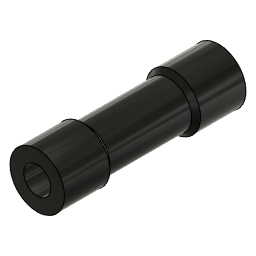
frame_assy (Autodesk Fusion 360 archive; units mm, degrees)
design "m3_standoff_20mm"
Autodesk Fusion 360 part; units mm, degrees
(part 1 of 5)
sketch "Sketch1" plane through (0, 0, 0) normal (0, 1, 0) x (1, 0, 0)
  line L0 (0, 0) -> (0, 20) construction
  line L1 (0, 20) -> (1.5, 20)
  line L2 (1.5, 20) -> (1.5, -8)
  line L3 (1.5, -8) -> (0, -8)
  line L4 (0, -8) -> (0, 20)
  line L5 (0, 20) -> (3, 20)
  line L6 (3, 20) -> (3, 15)
  line L7 (3, 15) -> (0, 15)
  line L8 (0, 15) -> (0, 20)
  line L9 (0, 0) -> (3, 0)
  line L10 (3, 0) -> (3, 5)
  line L11 (3, 5) -> (0, 5)
  line L12 (0, 5) -> (0, 0)
  line L13 (0, 15) -> (2.5, 15)
  line L14 (2.5, 15) -> (2.5, -3)
  line L15 (2.5, -3) -> (0, -3)
  line L16 (0, -3) -> (0, 15)
  dimension "d1" = 20
  dimension "d2" = 1.5
  dimension "d3" = 28
  dimension "d4" = 3
  dimension "d5" = 5
  dimension "d6" = 3
  dimension "d7" = 5
  dimension "d8" = 2.5
  constraint coincident L0.start L9.start
  constraint vertical L0
  constraint horizontal L1
  constraint vertical L2
  constraint horizontal L3
  constraint vertical L4
  constraint horizontal L5
  constraint vertical L6
  constraint horizontal L7
  constraint vertical L8
  constraint horizontal L9
  constraint vertical L10
  constraint horizontal L11
  constraint vertical L12
  constraint horizontal L13
  constraint vertical L14
  constraint horizontal L15
  constraint vertical L16
  measures "d1" distance of L0.start L0.end
  measures "d2" distance of L0.end L1.end
  measures "d3" distance of L0.end L3.end
  measures "d4" distance of L0.end L5.end
  measures "d5" distance of L0.end L7.end
  measures "d6" distance of L0.start L9.end
  measures "d7" distance of L0.start L11.end
  measures "d8" distance of L7.end L13.end
revolve "Revolve1" add sketch "Sketch1" angle 360 about axis through (0, 0, 3) along (0, 0, -1) contours L2 L5 L6 L7 L13 | L2 L7 L11 L13 L14 | L2 L9 L11 L14 | L9 L10 L11 L14
chamfer "Chamfer1" distance 0.5 angle 45 2 edges at (-2.3308, -0.904, -15) (-2.3308, -0.904, -5)

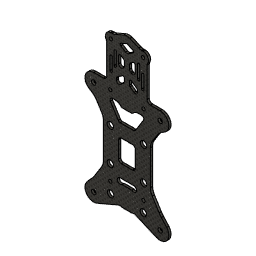
design "bottom_plate_2mm"
Autodesk Fusion 360 part; units mm, degrees
sketch "Sketch1" plane through (0, 0, 0) normal (0, 0, 1) x (1, 0, 0)
  line L0 (0, 26.674) -> (0, -149.1667) construction
  line L1 (30.5, -37.4) -> (-30.5, -37.4) construction
  line L2 (-30.5, -37.4) -> (-30.5, -124.4) construction
  line L3 (-30.5, -124.4) -> (30.5, -124.4) construction
  line L4 (30.5, -124.4) -> (30.5, -37.4) construction
  line L5 (30.5, -37.4) -> (-30.5, -124.4) construction
  line L6 (-30.5, -37.4) -> (30.5, -124.4) construction
  line L7 (-15.25, -63.8) -> (15.25, -63.8) construction
  line L8 (15.25, -63.8) -> (15.25, -94.3) construction
  line L9 (15.25, -94.3) -> (-15.25, -94.3) construction
  line L10 (-15.25, -94.3) -> (-15.25, -63.8) construction
  line L11 (-15.25, -63.8) -> (15.25, -94.3) construction
  line L12 (15.25, -63.8) -> (-15.25, -94.3) construction
  line L13 (5.15, -89.2) -> (-5.15, -89.2)
  line L14 (-7.65, -86.7) -> (-7.65, -71.4)
  line L15 (-5.15, -68.9) -> (5.15, -68.9)
  line L16 (7.65, -71.4) -> (7.65, -86.7)
  line L17 (7.65, -89.2) -> (-7.65, -68.9) construction
  line L18 (-7.65, -89.2) -> (7.65, -68.9) construction
  circle A0 centre (14.75, 5.1) radius 1.5
  line L19 (0, 0) -> (0, 7.5) construction
  line L20 (0, 7.5) -> (0, 13.8) construction
  line L21 (18.55, 0.8857) -> (18.55, -26.4)
  line L22 (14.75, 10.1) -> (0, 10.1)
  line L23 (21.55, -29.4) -> (30.5, -29.4)
  circle A1 centre (15.25, -63.8) radius 2.95
  circle A2 centre (15.25, -94.3) radius 2.95
  circle A3 centre (-15.25, -94.3) radius 2.95
  circle A4 centre (-15.25, -63.8) radius 2.95
  line L24 (12.25, 10.1) -> (0, 15.4402)
  circle A5 centre (15.25, -35.5) radius 1.5
  arc A6 (18.55, -26.4) -> (21.55, -29.4) centre (21.55, -26.4) ccw
  line L25 (30.5, -37.4) -> (30.5, -29.4) construction
  circle A7 centre (30.5, -37.4) radius 8
  circle A8 centre (30.5, -37.4) radius 2
  circle A9 centre (30.5, -124.4) radius 2
  circle A10 centre (30.5, -124.4) radius 8
  arc A11 (-5.15, -68.9) -> (-7.65, -71.4) centre (-5.15, -71.4) ccw
  arc A12 (7.65, -71.4) -> (5.15, -68.9) centre (5.15, -71.4) ccw
  arc A13 (5.15, -89.2) -> (7.65, -86.7) centre (5.15, -86.7) ccw
  arc A14 (-7.65, -86.7) -> (-5.15, -89.2) centre (-5.15, -86.7) ccw
  arc A15 (19, 2.4661) -> (14.75, 10.1) centre (14.75, 5.1) ccw
  arc A16 (14.75, 10.1) -> (18.55, 1.8504) centre (14.75, 5.1) ccw
  arc A17 (19, 2.4661) -> (18.55, 0.8857) centre (21.55, 0.8857) ccw
  line L26 (21.55, -98.0838) -> (21.55, -90.0777)
  line L27 (21.55, -90.0777) -> (21.55, -60.0565)
  line L28 (21.55, -60.0565) -> (30.7101, -45.3972)
  line L29 (21.55, -60.0565) -> (38.6049, -60.0565) construction
  line L30 (21.55, -98.0838) -> (30.5, -112.4068)
  line L31 (21.55, -98.0838) -> (38.4394, -98.0838) construction
  line L32 (30.5, -112.4068) -> (36.4601, -119.0636)
  line L33 (0, -123.6) -> (4.5, -123.6)
  line L34 (4.5, -123.6) -> (8.3, -123.6) construction
  arc A18 (8.3, -123.6) -> (4.5, -123.6) centre (6.4, -126.96) ccw
  line L35 (6.4, -123.1) -> (6.4, -123.6) construction
  line L36 (8.3, -123.6) -> (27.3521, -131.7546)
  line L37 (15.25, -94.3) -> (15.25, -108.3) construction
  circle A19 centre (15.25, -108.3) radius 1.5
  circle A20 centre (15, -118.1) radius 2.95
  arc A21 (-18.55, 1.8504) -> (-14.75, 10.1) centre (-14.75, 5.1) ccw
  line L38 (-21.55, -60.0565) -> (-30.7101, -45.3972)
  line L39 (-18.55, 0.8857) -> (-18.55, -26.4)
  circle A22 centre (-15.25, -35.5) radius 1.5
  circle A23 centre (-30.5, -37.4) radius 2
  line L40 (-14.75, 10.1) -> (0, 10.1)
  line L41 (0, 0) -> (0, 7.5) construction
  line L42 (-21.55, -90.0777) -> (-21.55, -60.0565)
  circle A24 centre (-14.75, 5.1) radius 1.5
  line L43 (-15.25, -63.8) -> (-15.25, -94.3) construction
  line L44 (-21.55, -29.4) -> (-30.5, -29.4)
  line L45 (-7.65, -89.2) -> (7.65, -68.9) construction
  line L46 (0, 7.5) -> (0, 13.8) construction
  arc A25 (-14.75, 10.1) -> (-19, 2.4661) centre (-14.75, 5.1) ccw
  line L47 (-30.5, -124.4) -> (-30.5, -37.4) construction
  line L48 (-21.55, -98.0838) -> (-30.5, -112.4068)
  line L49 (-12.25, 10.1) -> (0, 15.4402)
  arc A26 (-18.55, 0.8857) -> (-19, 2.4661) centre (-21.55, 0.8857) ccw
  line L50 (0, -123.6) -> (-4.5, -123.6)
  circle A27 centre (-15.25, -63.8) radius 2.95
  circle A28 centre (-30.5, -37.4) radius 8
  arc A29 (-21.55, -29.4) -> (-18.55, -26.4) centre (-21.55, -26.4) ccw
  line L51 (-30.5, -37.4) -> (-30.5, -29.4) construction
  line L52 (-21.55, -98.0838) -> (-38.4394, -98.0838) construction
  circle A30 centre (-15.25, -94.3) radius 2.95
  line L53 (5.15, -68.9) -> (-5.15, -68.9)
  line L54 (-6.4, -123.1) -> (-6.4, -123.6) construction
  arc A31 (-5.15, -68.9) -> (-7.65, -71.4) centre (-5.15, -71.4) ccw
  line L55 (-21.55, -98.0838) -> (-21.55, -90.0777)
  line L56 (-7.65, -71.4) -> (-7.65, -86.7)
  arc A32 (7.65, -71.4) -> (5.15, -68.9) centre (5.15, -71.4) ccw
  arc A33 (5.15, -89.2) -> (7.65, -86.7) centre (5.15, -86.7) ccw
  arc A34 (-7.65, -86.7) -> (-5.15, -89.2) centre (-5.15, -86.7) ccw
  line L57 (7.65, -86.7) -> (7.65, -71.4)
  line L58 (7.65, -89.2) -> (-7.65, -68.9) construction
  line L59 (-21.55, -60.0565) -> (-38.6049, -60.0565) construction
  line L60 (-8.3, -123.6) -> (-27.3521, -131.7546)
  line L61 (-15.25, -94.3) -> (-15.25, -108.3) construction
  circle A35 centre (-15, -118.1) radius 2.95
  line L62 (-30.5, -112.4068) -> (-36.4601, -119.0636)
  line L63 (-4.5, -123.6) -> (-8.3, -123.6) construction
  circle A36 centre (-30.5, -124.4) radius 8
  arc A37 (-4.5, -123.6) -> (-8.3, -123.6) centre (-6.4, -126.96) ccw
  circle A38 centre (-15.25, -108.3) radius 1.5
  circle A39 centre (-30.5, -124.4) radius 2
  line L64 (-5.15, -89.2) -> (5.15, -89.2)
  point P0 (0, -80.9)
  point P1 (0, -79.05)
  point P2 (0, -79.05)
  point P3 (18.55, -29.4)
  point P4 (0, -149.1667)
  point P5 (0, -79.05)
  point P6 (0, 26.674)
  point P7 (-18.55, -29.4)
  point P8 (0, -79.05)
  point P9 (0, -80.9)
  dimension "d1" = 61
  dimension "d2" = 87
  dimension "d3" = 30.5
  dimension "d4" = 30.5
  dimension "d7" = 15.3
  dimension "d8" = 20.3
  dimension "d9" = 68.9
  dimension "d10" = 3
  dimension "d11" = 14.75
  dimension "d14" = 7.5
  dimension "d15" = 6.3
  dimension "d17" = 10
  dimension "d18" = 18.55
  dimension "d19" = 39.5
  dimension "d20" = 5.9
  dimension "d21" = 8.7
  dimension "d22" = 2.5
  dimension "d24" = 3
  dimension "d25" = 15.25
  dimension "d26" = 40.6
  dimension "d27" = 3
  dimension "d28" = 8
  dimension "d29" = 4
  dimension "d30" = 16
  dimension "d31" = 2.5
  dimension "d32" = 3
  dimension "d33" = 21.55
  dimension "d34" = 58
  dimension "d35" = 58
  dimension "d36" = 34.4
  dimension "d37" = 3.8
  dimension "d38" = 4.5
  dimension "d39" = 0.5
  dimension "d41" = 72.8
  dimension "d42" = 15
  dimension "d43" = 23.8
  constraint vertical L0
  constraint horizontal L1
  constraint perpendicular L1 L2
  constraint parallel L1 L3
  constraint parallel L2 L4
  constraint coincident L5 P9
  constraint coincident L6 P9
  constraint coincident L0 P9
  constraint horizontal L7
  constraint perpendicular L7 L8
  constraint parallel L7 L9
  constraint parallel L8 L10
  constraint coincident L11 P8
  constraint coincident L12 P8
  constraint coincident L0 P8
  constraint horizontal L13
  constraint perpendicular L13 L14
  constraint parallel L13 L15
  constraint parallel L14 L16
  constraint coincident L17 P8
  constraint coincident L18 P8
  constraint coincident P8 P5
  constraint coincident L19.start L41.start
  constraint parallel L0 L19
  constraint parallel L0 L20
  constraint concentric A0 A15
  constraint parallel L20 L21
  constraint coincident L0 L22.end
  constraint horizontal L22
  constraint perpendicular L21 L23
  constraint coincident L7.end L8.start
  constraint coincident L8.end L9.start
  constraint coincident L9.end L10.start
  constraint coincident L7.start L10.end
  constraint equal A3 A4
  constraint equal A2 A3
  constraint equal A1 A2
  constraint tangent L22 A15
  constraint coincident L22 L24.start
  constraint coincident L0 L24.end
  constraint coincident P3 L21
  constraint coincident P3 L23
  constraint tangent L21 A6
  constraint tangent L23 A6
  constraint coincident L23 L25.end
  constraint perpendicular L23 L25
  constraint coincident L1.start L4.end
  constraint coincident L23.end A7
  constraint concentric A7 A8
  constraint coincident L3.end L4.start
  constraint concentric A9 A10
  constraint equal A8 A9
  constraint coincident L17.end L15
  constraint coincident L17.end L14
  constraint tangent L15 A11
  constraint tangent L14 A11
  constraint coincident L18.end L15
  constraint coincident L18.end L16
  constraint tangent L15 A12
  constraint tangent L16 A12
  constraint equal A11 A12
  constraint coincident L17.start L16
  constraint coincident L17.start L13
  constraint tangent L16 A13
  constraint tangent L13 A13
  constraint equal A11 A13
  constraint coincident L18.start L13
  constraint coincident L18.start L14
  constraint tangent L13 A14
  constraint tangent L14 A14
  constraint equal A11 A14
  constraint concentric A15 A16
  constraint coincident A16.end L21
  constraint tangent A15 A17
  constraint tangent L21 A17
  constraint parallel L4 L26
  constraint parallel L4 L27
  constraint horizontal L29
  constraint coincident L27 L28.start
  constraint coincident A7 L28.end
  constraint horizontal L31
  constraint coincident L26 L30.start
  constraint coincident L4 L30.end
  constraint coincident A10 L32.end
  constraint tangent A10 L32
  constraint coincident L0 L33.start
  constraint perpendicular L0 L33
  constraint perpendicular L0 L34
  constraint midpoint A18 L35.start
  constraint midpoint L34 L35.end
  constraint coincident A10 L36.end
  constraint tangent A10 L36
  constraint perpendicular L9 L37
  constraint coincident L37.end A19.centre
  constraint equal A5 A19
  constraint equal A2 A20
  constraint symmetric L19.start L0 L41.start
  constraint symmetric P6 L0 L0.start
  constraint symmetric P4 L0 L0.end
  constraint symmetric L0 L1.start L1.end
  constraint symmetric L0 L3.end L2.end
  constraint symmetric L0 P9 P0
  constraint symmetric L0 L7.end L7.start
  constraint symmetric L0 L8.end L9.end
  constraint symmetric L0 P8 P5
  constraint symmetric L0 L17.start L18.start
  constraint symmetric L0 L18.start L17.start
  constraint symmetric L0 L17.end L18.end
  constraint symmetric L0 L18.end L17.end
  constraint symmetric L0 A0 A24
  constraint symmetric L0 L19.start L41.start
  constraint symmetric L0 L19.end L20.start
  constraint symmetric L0 L20.end L46.end
  constraint symmetric L0 A16.end A21.start
  constraint symmetric L0 P3 P7
  constraint symmetric L0 L22.start A21.end
  constraint symmetric L0 L22.end L40.end
  constraint symmetric L0 A1 A27
  constraint symmetric L0 A2 A30
  constraint symmetric L0 L24.start L49.start
  constraint symmetric L0 L24.end L49.end
  constraint symmetric L0 A5 A22
  constraint symmetric L0 L21.end L39.end
  constraint symmetric L0 L23.start L44.start
  constraint symmetric L0 A6 A29
  constraint symmetric L0 L23.end L44.end
  constraint symmetric L0 A7 A28
  constraint symmetric L0 A8 A23
  constraint symmetric L0 A9 A39
  constraint symmetric L0 A10 A36
  constraint symmetric L0 L15.start L15.end
  constraint symmetric L0 L14.end L16.start
  constraint symmetric L0 A11 A32
  constraint symmetric L0 L15.end L15.start
  constraint symmetric L0 L16.start L14.end
  constraint symmetric L0 A12 A31
  constraint symmetric L0 L16.end L14.start
  constraint symmetric L0 L13.start L13.end
  constraint symmetric L0 A13 A34
  constraint symmetric L0 L13.end L13.start
  constraint symmetric L0 L14.start L16.end
  constraint symmetric L0 A14 A33
  constraint symmetric L0 A15 A25
  constraint symmetric L0 A16 A21
  constraint symmetric L0 L21.start L39.start
  constraint symmetric L0 A15.start A25.end
  constraint symmetric L0 A17 A26
  constraint symmetric L0 L26.end L42.start
  constraint symmetric L0 L27.end L38.start
  constraint symmetric L0 L28.end L38.end
  constraint symmetric L0 L29.end L59.end
  constraint symmetric L0 L26.start L48.start
  constraint symmetric L0 L30.end L48.end
  constraint symmetric L0 L31.end L52.end
  constraint symmetric L0 L32.end L62.end
  constraint symmetric L0 L33.start L50.start
  constraint symmetric L0 L33.end L50.end
  constraint symmetric L0 L34.end L60.start
  constraint symmetric L0 A18 A37
  constraint symmetric L0 L35.start L54.start
  constraint symmetric L0 L35.end L54.end
  constraint symmetric L0 L36.end L60.end
  constraint symmetric L0 L37.end L61.end
  constraint symmetric L0 A19 A38
  constraint symmetric L0 A20 A35
  measures "d1" distance of L2.end L3.end
  measures "d2" distance of L1.end L2.end
  measures "d3" distance of L8.end L9.end
  measures "d4" distance of L7.end L8.end
  measures "d7" distance of L17.end L18.end
  measures "d8" distance of L18.start L17.end
  measures "d9" distance of L19.start L15
  measures "d10" diameter of A0
  measures "d11" distance of L0 A0.centre
  measures "d14" distance of L19.start L19.end
  measures "d15" distance of L19.end L20.end
  measures "d17" diameter of A15
  measures "d18" distance of L0 L21
  measures "d19" distance of P3 L22
  measures "d20" diameter of A1
  measures "d21" vertical distance of L20.end A0.centre
  measures "d22" distance of L22.start L24.start
  measures "d24" diameter of A5
  measures "d25" distance of L0 A5.centre
  measures "d26" vertical distance of A0.centre A5.centre
  measures "d27" radius of A6
  measures "d28" distance of L1.start L23.end
  measures "d29" diameter of A8
  measures "d30" diameter of A10
  measures "d31" radius of A11
  measures "d32" radius of A17
  measures "d33" distance of L0 L27
  measures "d34" angle of L28 L29
  measures "d35" angle of L30 L31
  measures "d36" distance of L13 L33
  measures "d37" distance of L33.end L34.end
  measures "d38" distance of L33.start L33.end
  measures "d39" distance of L35.start L35.end
  measures "d41" distance of A5.centre L37.end
  measures "d42" distance of L0 A20.centre
  measures "d43" vertical distance of L8.end A20.centre
extrude "Extrude1" add sketch "Sketch1" along normal blind 2
fillet "Fillet1" radius 15 2 edges at (30.7101, -45.3972, 1) (-30.7101, -45.3972, 1)
fillet "Fillet2" radius 20 2 edges at (30.5, -112.4068, 1) (-30.5, -112.4068, 1)
fillet "Fillet3" radius 11 4 edges at (21.55, -98.0838, 1) (-21.55, -98.0838, 1) (21.55, -60.0565, 1) (-21.55, -60.0565, 1)
fillet "Fillet4" radius 7 3 edges at (12.25, 10.1, 1) (-12.25, 10.1, 1) (0, 15.4402, 1)
sketch "Sketch2" plane through (0, 0, 2) normal (0, 0, 1) x (1, 0, 0)
  arc A0 (2.7973, 14.2208) -> (-2.7973, 14.2208) centre (0, 7.804) ccw
  line L0 (-2.7973, 14.2208) -> (-10.9121, 10.6832)
  arc A1 (-13.7095, 10.1) -> (-10.9121, 10.6832) centre (-13.7095, 17.1) ccw
  line L1 (-13.7095, 10.1) -> (-14.75, 10.1)
  arc A2 (-14.75, 10.1) -> (-19, 2.4661) centre (-14.75, 5.1) ccw
  arc A3 (-18.55, 0.8857) -> (-19, 2.4661) centre (-21.55, 0.8857) ccw
  line L2 (-18.55, 0.8857) -> (-18.55, -26.4)
  arc A4 (-21.55, -29.4) -> (-18.55, -26.4) centre (-21.55, -26.4) ccw
  line L3 (-21.55, -29.4) -> (-30.5, -29.4)
  arc A5 (-30.5, -29.4) -> (-33.9547, -44.6156) centre (-30.5, -37.4) ccw
  arc A6 (-27.7114, -50.1961) -> (-33.9547, -44.6156) centre (-40.4322, -58.1449) ccw
  line L4 (-27.7114, -50.1961) -> (-23.2215, -57.3816)
  arc A7 (-21.55, -63.2107) -> (-23.2215, -57.3816) centre (-32.55, -63.2107) ccw
  line L5 (-21.55, -63.2107) -> (-21.55, -94.9296)
  arc A8 (-23.2215, -100.7587) -> (-21.55, -94.9296) centre (-32.55, -94.9296) ccw
  line L6 (-23.2215, -100.7587) -> (-29.5877, -110.9469)
  arc A9 (-31.6483, -113.6894) -> (-29.5877, -110.9469) centre (-46.5487, -100.3485) ccw
  line L7 (-31.6483, -113.6894) -> (-36.4601, -119.0636)
  arc A10 (-36.4601, -119.0636) -> (-27.3521, -131.7546) centre (-30.5, -124.4) ccw
  line L8 (-27.3521, -131.7546) -> (-8.3, -123.6)
  arc A11 (-4.5, -123.6) -> (-8.3, -123.6) centre (-6.4, -126.96) ccw
  line L9 (-4.5, -123.6) -> (4.5, -123.6)
  arc A12 (8.3, -123.6) -> (4.5, -123.6) centre (6.4, -126.96) ccw
  line L10 (8.3, -123.6) -> (27.3521, -131.7546)
  arc A13 (27.3521, -131.7546) -> (36.4601, -119.0636) centre (30.5, -124.4) ccw
  line L11 (36.4601, -119.0636) -> (31.6483, -113.6894)
  arc A14 (29.5877, -110.9469) -> (31.6483, -113.6894) centre (46.5487, -100.3485) ccw
  line L12 (29.5877, -110.9469) -> (23.2215, -100.7587)
  arc A15 (21.55, -94.9296) -> (23.2215, -100.7587) centre (32.55, -94.9296) ccw
  line L13 (21.55, -94.9296) -> (21.55, -63.2107)
  arc A16 (23.2215, -57.3816) -> (21.55, -63.2107) centre (32.55, -63.2107) ccw
  line L14 (23.2215, -57.3816) -> (27.7114, -50.1961)
  arc A17 (33.9547, -44.6156) -> (27.7114, -50.1961) centre (40.4322, -58.1449) ccw
  arc A18 (33.9547, -44.6156) -> (30.5, -29.4) centre (30.5, -37.4) ccw
  line L15 (30.5, -29.4) -> (21.55, -29.4)
  arc A19 (18.55, -26.4) -> (21.55, -29.4) centre (21.55, -26.4) ccw
  line L16 (18.55, -26.4) -> (18.55, 0.8857)
  arc A20 (19, 2.4661) -> (18.55, 0.8857) centre (21.55, 0.8857) ccw
  arc A21 (19, 2.4661) -> (14.75, 10.1) centre (14.75, 5.1) ccw
  line L17 (14.75, 10.1) -> (13.7095, 10.1)
  arc A22 (10.9121, 10.6832) -> (13.7095, 10.1) centre (13.7095, 17.1) ccw
  line L18 (10.9121, 10.6832) -> (2.7973, 14.2208)
  circle A23 centre (14.75, 5.1) radius 1.5
  circle A24 centre (15.25, -63.8) radius 2.95
  circle A25 centre (15.25, -35.5) radius 1.5
  circle A26 centre (15.25, -94.3) radius 2.95
  circle A27 centre (30.5, -37.4) radius 2
  circle A28 centre (30.5, -124.4) radius 2
  circle A29 centre (15.25, -108.3) radius 1.5
  circle A30 centre (15, -118.1) radius 2.95
  circle A31 centre (-15.25, -35.5) radius 1.5
  circle A32 centre (-30.5, -37.4) radius 2
  circle A33 centre (-14.75, 5.1) radius 1.5
  circle A34 centre (-15.25, -63.8) radius 2.95
  circle A35 centre (-15.25, -94.3) radius 2.95
  circle A36 centre (-15, -118.1) radius 2.95
  circle A37 centre (-15.25, -108.3) radius 1.5
  circle A38 centre (-30.5, -124.4) radius 2
  line L19 (5.15, -89.2) -> (-5.15, -89.2)
  arc A39 (-7.65, -86.7) -> (-5.15, -89.2) centre (-5.15, -86.7) ccw
  line L20 (-7.65, -86.7) -> (-7.65, -71.4)
  arc A40 (-5.15, -68.9) -> (-7.65, -71.4) centre (-5.15, -71.4) ccw
  line L21 (-5.15, -68.9) -> (5.15, -68.9)
  arc A41 (7.65, -71.4) -> (5.15, -68.9) centre (5.15, -71.4) ccw
  line L22 (7.65, -71.4) -> (7.65, -86.7)
  arc A42 (5.15, -89.2) -> (7.65, -86.7) centre (5.15, -86.7) ccw
  line L23 (5.4482, 6.3017) -> (0.3197, 8.5373)
  arc A43 (0.3197, 8.5373) -> (-0.3197, 8.5373) centre (0, 7.804) ccw
  line L24 (-0.3197, 8.5373) -> (-5.4482, 6.3017)
  line L25 (-1.3481, 1.3661) -> (-5.6227, 4.1031)
  line L26 (0, 26.674) -> (0, -149.1667)
  line L27 (1.3481, 1.3661) -> (5.6227, 4.1031)
  line L28 (13.55, -8.5) -> (13.55, -20.5)
  arc A44 (13.55, -20.5) -> (15.55, -20.5) centre (14.55, -20.5) ccw
  line L29 (15.55, -20.5) -> (15.55, -8.5)
  arc A45 (15.55, -8.5) -> (13.55, -8.5) centre (14.55, -8.5) ccw
  line L30 (14.55, -7.5) -> (14.55, -21.5) construction
  line L31 (18.55, 0.8857) -> (18.55, -26.4)
  circle A46 centre (15.25, -35.5) radius 1.5
  line L32 (9.75, -2.5) -> (9.75, -14.5)
  arc A47 (9.75, -14.5) -> (11.75, -14.5) centre (10.75, -14.5) ccw
  line L33 (11.75, -14.5) -> (11.75, -2.5)
  arc A48 (11.75, -2.5) -> (9.75, -2.5) centre (10.75, -2.5) ccw
  line L34 (10.75, -1.5) -> (10.75, -15.5) construction
  line L35 (2.35, -6.7029) -> (2.35, -10.5206)
  line L36 (7.55, -4.3629) -> (7.55, -11.0338)
  line L37 (3.3637, -4.8501) -> (5.7029, -3.3523)
  line L38 (3.3622, -12.3724) -> (4.1622, -12.8855)
  arc A49 (3.3637, -4.8501) -> (2.35, -6.7029) centre (4.55, -6.7029) ccw
  arc A50 (2.35, -10.5206) -> (3.3622, -12.3724) centre (4.55, -10.5206) ccw
  arc A51 (4.1622, -12.8855) -> (7.55, -11.0338) centre (5.35, -11.0338) ccw
  arc A52 (7.55, -4.3629) -> (5.7029, -3.3523) centre (6.35, -4.3629) ccw
  line L39 (2.35, -19.8578) -> (2.35, -23.0931)
  line L40 (9.65, -23.8089) -> (9.65, -25.2396)
  line L41 (4.253, -18.8853) -> (8.8217, -22.188)
  line L42 (2.818, -24.044) -> (6.43, -26.8244)
  arc A53 (4.253, -18.8853) -> (2.35, -19.8578) centre (3.55, -19.8578) ccw
  arc A54 (2.35, -23.0931) -> (2.818, -24.044) centre (3.55, -23.0931) ccw
  arc A55 (6.43, -26.8244) -> (9.65, -25.2396) centre (7.65, -25.2396) ccw
  arc A56 (9.65, -23.8089) -> (8.8217, -22.188) centre (7.65, -23.8089) ccw
  arc A57 (-5.4482, 6.3017) -> (-5.6227, 4.1031) centre (-4.9486, 5.1558) ccw
  arc A58 (5.6227, 4.1031) -> (5.4482, 6.3017) centre (4.9486, 5.1558) ccw
  arc A59 (-1.3481, 1.3661) -> (1.3481, 1.3661) centre (0, 3.4715) ccw
  line L43 (-5.15, -68.9) -> (5.15, -68.9)
  line L44 (0, -57.15) -> (6.189, -57.15)
  line L45 (0, -44.45) -> (4.8532, -44.45)
  line L46 (7.8851, -56.2098) -> (15.1961, -44.5098)
  line L47 (7.2976, -57.15) -> (28.8558, -57.15) construction
  line L48 (10.3384, -41.45) -> (13.5, -41.45)
  line L49 (4.8532, -44.45) -> (6.0958, -43.2074)
  line L50 (4.8532, -44.45) -> (9.5326, -44.45) construction
  arc A60 (10.3384, -41.45) -> (6.0958, -43.2074) centre (10.3384, -47.45) ccw
  arc A61 (15.1961, -44.5098) -> (13.5, -41.45) centre (13.5, -43.45) ccw
  arc A62 (6.189, -57.15) -> (7.8851, -56.2098) centre (6.189, -55.15) ccw
  line L51 (0, -100.95) -> (6.6112, -100.95)
  line L52 (0, -105.45) -> (4.5, -105.45)
  line L53 (4.5, -123.6) -> (4.5, -105.45) construction
  line L54 (8.0447, -101.6962) -> (8.3897, -102.1889)
  line L55 (7.5222, -100.95) -> (12.5593, -100.95) construction
  arc A63 (4.5, -105.45) -> (8.3897, -102.1889) centre (6.3028, -103.6501) ccw
  arc A64 (8.0447, -101.6962) -> (6.6112, -100.95) centre (6.6112, -102.7) ccw
  line L56 (0, -105.45) -> (-4.5, -105.45)
  line L57 (-8.0447, -101.6962) -> (-8.3897, -102.1889)
  arc A65 (-8.3897, -102.1889) -> (-4.5, -105.45) centre (-6.3028, -103.6501) ccw
  arc A66 (-6.6112, -100.95) -> (-8.0447, -101.6962) centre (-6.6112, -102.7) ccw
  line L58 (0, -100.95) -> (-6.6112, -100.95)
  line L59 (0, -44.45) -> (-4.8532, -44.45)
  arc A67 (-6.0958, -43.2074) -> (-10.3384, -41.45) centre (-10.3384, -47.45) ccw
  line L60 (-7.8851, -56.2098) -> (-15.1961, -44.5098)
  line L61 (-10.3384, -41.45) -> (-13.5, -41.45)
  line L62 (0, -57.15) -> (-6.189, -57.15)
  line L63 (-4.8532, -44.45) -> (-9.5326, -44.45) construction
  arc A68 (-7.8851, -56.2098) -> (-6.189, -57.15) centre (-6.189, -55.15) ccw
  line L64 (-4.8532, -44.45) -> (-6.0958, -43.2074)
  arc A69 (-13.5, -41.45) -> (-15.1961, -44.5098) centre (-13.5, -43.45) ccw
  arc A70 (-5.7029, -3.3523) -> (-7.55, -4.3629) centre (-6.35, -4.3629) ccw
  arc A71 (-13.55, -8.5) -> (-15.55, -8.5) centre (-14.55, -8.5) ccw
  arc A72 (-8.8217, -22.188) -> (-9.65, -23.8089) centre (-7.65, -23.8089) ccw
  arc A73 (-9.65, -25.2396) -> (-6.43, -26.8244) centre (-7.65, -25.2396) ccw
  line L65 (-9.65, -23.8089) -> (-9.65, -25.2396)
  line L66 (-13.55, -8.5) -> (-13.55, -20.5)
  line L67 (-3.3637, -4.8501) -> (-5.7029, -3.3523)
  arc A74 (-15.55, -20.5) -> (-13.55, -20.5) centre (-14.55, -20.5) ccw
  arc A75 (-7.55, -11.0338) -> (-4.1622, -12.8855) centre (-5.35, -11.0338) ccw
  arc A76 (-3.3622, -12.3724) -> (-2.35, -10.5206) centre (-4.55, -10.5206) ccw
  line L68 (-15.55, -20.5) -> (-15.55, -8.5)
  line L69 (-10.75, -1.5) -> (-10.75, -15.5) construction
  line L70 (-4.253, -18.8853) -> (-8.8217, -22.188)
  line L71 (-14.55, -7.5) -> (-14.55, -21.5) construction
  line L72 (-2.818, -24.044) -> (-6.43, -26.8244)
  line L73 (-2.35, -19.8578) -> (-2.35, -23.0931)
  line L74 (-2.35, -6.7029) -> (-2.35, -10.5206)
  arc A77 (-2.35, -19.8578) -> (-4.253, -18.8853) centre (-3.55, -19.8578) ccw
  line L75 (-7.55, -4.3629) -> (-7.55, -11.0338)
  line L76 (-9.75, -2.5) -> (-9.75, -14.5)
  line L77 (-3.3622, -12.3724) -> (-4.1622, -12.8855)
  line L78 (-11.75, -14.5) -> (-11.75, -2.5)
  arc A78 (-2.35, -6.7029) -> (-3.3637, -4.8501) centre (-4.55, -6.7029) ccw
  arc A79 (-11.75, -14.5) -> (-9.75, -14.5) centre (-10.75, -14.5) ccw
  arc A80 (-9.75, -2.5) -> (-11.75, -2.5) centre (-10.75, -2.5) ccw
  arc A81 (-2.818, -24.044) -> (-2.35, -23.0931) centre (-3.55, -23.0931) ccw
  point P0 (15.25, -35.5)
  point P1 (-7.5222, -100.95)
  point P2 (-7.2976, -57.15)
  point P3 (-18.55, -26.4)
  point P4 (-18.55, -26.4)
  dimension "d55" = 2
  dimension "d56" = 14
  dimension "d57" = 3
  dimension "d58" = 14
  dimension "d59" = 2
  dimension "d60" = 14
  dimension "d61" = 1.8
  dimension "d62" = 6
  dimension "d63" = 2.35
  dimension "d64" = 5.2
  dimension "d65" = 2.2
  dimension "d66" = 1.2
  dimension "d67" = 2.35
  dimension "d68" = 7.3
  dimension "d69" = 1.2
  dimension "d70" = 2
  dimension "d71" = 1.25
  dimension "d72" = 1.25
  dimension "d73" = 2.5
  dimension "d74" = 11.75
  dimension "d75" = 12.7
  dimension "d76" = 58
  dimension "d77" = 3
  dimension "d78" = 45
  dimension "d79" = 6
  dimension "d80" = 2
  dimension "d81" = 2
  dimension "d82" = 11.75
  dimension "d83" = 4.5
  dimension "d84" = 55
  dimension "d85" = 1.75
  dimension "d86" = 13.5
  constraint tangent L28 A44
  constraint tangent A44 L29
  constraint parallel L28 L29
  constraint tangent L29 A45
  constraint tangent L28 A45
  constraint midpoint A45 L30.start
  constraint midpoint A44 L30.end
  constraint vertical L30
  constraint tangent L32 A47
  constraint tangent A47 L33
  constraint parallel L32 L33
  constraint tangent L33 A48
  constraint tangent L32 A48
  constraint midpoint A48 L34.start
  constraint midpoint A47 L34.end
  constraint vertical L34
  constraint parallel L32 L35
  constraint parallel L34 L36
  constraint parallel L27 L37
  constraint tangent L37 A49
  constraint tangent L35 A49
  constraint tangent L35 A50
  constraint tangent L38 A50
  constraint equal A49 A50
  constraint tangent L38 A51
  constraint tangent L36 A51
  constraint equal A49 A51
  constraint tangent L37 A52
  constraint tangent L36 A52
  constraint vertical L39
  constraint vertical L40
  constraint tangent L41 A53
  constraint tangent L39 A53
  constraint tangent L42 A54
  constraint tangent L39 A54
  constraint equal A53 A54
  constraint tangent L42 A55
  constraint tangent L40 A55
  constraint tangent L40 A56
  constraint tangent L41 A56
  constraint equal A55 A56
  constraint concentric A0 A43
  constraint tangent L23 A43
  constraint tangent A43 L24
  constraint tangent L25 A57
  constraint tangent L24 A57
  constraint tangent L23 A58
  constraint tangent L27 A58
  constraint tangent L27 A59
  constraint tangent L25 A59
  constraint coincident L26 L44.start
  constraint perpendicular L26 L44
  constraint coincident L26 L45.start
  constraint perpendicular L26 L45
  constraint horizontal L47
  constraint horizontal L48
  constraint horizontal L50
  constraint tangent L48 A60
  constraint tangent L49 A60
  constraint tangent L46 A61
  constraint tangent L48 A61
  constraint coincident L47.start L46
  constraint coincident L47.start L44
  constraint tangent L46 A62
  constraint tangent L44 A62
  constraint coincident L26 L51.start
  constraint perpendicular L26 L51
  constraint coincident L26 L52.start
  constraint perpendicular L26 L52
  constraint coincident L9.end A12.end
  constraint vertical L53
  constraint horizontal L55
  constraint tangent L54 A63
  constraint coincident L55.start L54
  constraint coincident L55.start L51
  constraint tangent L54 A64
  constraint tangent L51 A64
  constraint symmetric L26 L51.start L58.start
  constraint symmetric L26 L55.start P1
  constraint symmetric L26 L52.start L56.start
  constraint symmetric L26 L52.end L56.end
  constraint symmetric L26 L54.end L57.end
  constraint symmetric L26 A63 A65
  constraint symmetric L26 L54.start L57.start
  constraint symmetric L26 L51.end A66.start
  constraint symmetric L26 A64 A66
  constraint symmetric L26 L44.start L62.start
  constraint symmetric L26 L47.start P2
  constraint symmetric L26 L45.start L59.start
  constraint symmetric L26 L45.end L59.end
  constraint symmetric L26 L50.end L63.end
  constraint symmetric L26 L48.start A67.end
  constraint symmetric L26 L49.end A67.start
  constraint symmetric L26 A60 A67
  constraint symmetric L26 L46.end L60.end
  constraint symmetric L26 L48.end L61.end
  constraint symmetric L26 A61 A69
  constraint symmetric L26 L46.start L60.start
  constraint symmetric L26 L44.end L62.end
  constraint symmetric L26 A62 A68
  constraint symmetric A19.start L26 P4
  constraint symmetric L26 L28.start A71.start
  constraint symmetric L26 L28.end L66.end
  constraint symmetric L26 A44.end A74.start
  constraint symmetric L26 L29.end A71.end
  constraint symmetric L26 A44 A74
  constraint symmetric L26 A45 A71
  constraint symmetric L26 L30.start L71.start
  constraint symmetric L26 L30.end L71.end
  constraint symmetric L26 A19.start P4
  constraint symmetric L26 L32.start L76.start
  constraint symmetric L26 L32.end L76.end
  constraint symmetric L26 A47.end L78.start
  constraint symmetric L26 L33.end L78.end
  constraint symmetric L26 A47 A79
  constraint symmetric L26 A48 A80
  constraint symmetric L26 L34.start L69.start
  constraint symmetric L26 L34.end L69.end
  constraint symmetric L26 L37.start L67.start
  constraint symmetric L26 L35.start L74.start
  constraint symmetric L26 A49 A78
  constraint symmetric L26 L35.end A76.end
  constraint symmetric L26 L38.start A76.start
  constraint symmetric L26 A50 A76
  constraint symmetric L26 L38.end A75.end
  constraint symmetric L26 L36.end A75.start
  constraint symmetric L26 A51 A75
  constraint symmetric L26 L37.end A70.start
  constraint symmetric L26 L36.start A70.end
  constraint symmetric L26 A52 A70
  constraint symmetric L26 L41.start L70.start
  constraint symmetric L26 L39.start L73.start
  constraint symmetric L26 A53 A77
  constraint symmetric L26 L42.start L72.start
  constraint symmetric L26 L39.end L73.end
  constraint symmetric L26 A54 A81
  constraint symmetric L26 L42.end A73.end
  constraint symmetric L26 L40.end A73.start
  constraint symmetric L26 A55 A73
  constraint symmetric L26 L40.start A72.end
  constraint symmetric L26 L41.end A72.start
  constraint symmetric L26 A56 A72
  measures "d55" diameter of A44
  measures "d56" distance of L30.start L30.end
  measures "d57" distance of L29 L31
  measures "d58" vertical distance of L30.end P0
  measures "d59" diameter of A47
  measures "d60" distance of L34.start L34.end
  measures "d61" distance of L28 L33
  measures "d62" vertical distance of L30.end L34.end
  measures "d63" distance of L26 L35
  measures "d64" distance of L35 L36
  measures "d65" radius of A49
  measures "d66" radius of A52
  measures "d67" distance of L26 L39
  measures "d68" distance of L39 L40
  measures "d69" radius of A53
  measures "d70" radius of A55
  measures "d71" radius of A57
  measures "d72" radius of A58
  measures "d73" radius of A59
  measures "d74" distance of L43 L44
  measures "d75" distance of L44 L45
  measures "d76" angle of L46 L47
  measures "d77" distance of L45 L48
  measures "d78" angle of L49 L50
  measures "d79" radius of A60
  measures "d80" radius of A61
  measures "d81" radius of A62
  measures "d82" distance of L19 L51
  measures "d83" distance of L51 L52
  measures "d84" angle of L54 L55
  measures "d85" radius of A64
  measures "d86" distance of L26 A61.centre
extrude "Extrude2" cut sketch "Sketch2" against normal blind 2 contours A43 L24 L25 L26 A57 A59 | L23 A43 L26 L27 A58 A59 | L26 L44 L45 L46 L48 L49 A60 A61 A62 | L26 L59 A67 L60 L61 L62 A68 L64 A69 | L26 L51 L52 L54 A63 A64 | L26 L56 L57 A65 A66 L58 | L28 A44 L29 A45 | L32 A47 L33 A48 | L35 L36 L37 L38 A49 A50 A51 A52 | L39 L40 L41 L42 A53 A54 A55 A56 | A70 L67 A75 A76 L74 L75 L77 A78 | A71 L66 A74 L68 | A72 A73 L65 L70 L72 L73 A77 A81 | L76 L78 A79 A80
sketch "Sketch3" plane through (0, 0, 0) normal (0, 0, 1) x (1, 0, 0)
  line L0 (13.55, -20.5) -> (13.55, -8.5)
  arc A0 (15.55, -8.5) -> (13.55, -8.5) centre (14.55, -8.5) ccw
  line L1 (15.55, -8.5) -> (15.55, -20.5)
  arc A1 (13.55, -20.5) -> (15.55, -20.5) centre (14.55, -20.5) ccw
  line L2 (-8.8217, -22.188) -> (-4.253, -18.8853)
  arc A2 (-2.35, -19.8578) -> (-4.253, -18.8853) centre (-3.55, -19.8578) ccw
  line L3 (-2.35, -19.8578) -> (-2.35, -23.0931)
  arc A3 (-2.818, -24.044) -> (-2.35, -23.0931) centre (-3.55, -23.0931) ccw
  line L4 (-2.818, -24.044) -> (-6.43, -26.8244)
  arc A4 (-9.65, -25.2396) -> (-6.43, -26.8244) centre (-7.65, -25.2396) ccw
  line L5 (-9.65, -25.2396) -> (-9.65, -23.8089)
  arc A5 (-8.8217, -22.188) -> (-9.65, -23.8089) centre (-7.65, -23.8089) ccw
  line L6 (5.6227, 4.1031) -> (1.3481, 1.3661)
  arc A6 (-1.3481, 1.3661) -> (1.3481, 1.3661) centre (0, 3.4715) ccw
  line L7 (-1.3481, 1.3661) -> (-5.6227, 4.1031)
  arc A7 (-5.4482, 6.3017) -> (-5.6227, 4.1031) centre (-4.9486, 5.1558) ccw
  line L8 (-5.4482, 6.3017) -> (-0.3197, 8.5373)
  arc A8 (0.3197, 8.5373) -> (-0.3197, 8.5373) centre (0, 7.804) ccw
  line L9 (0.3197, 8.5373) -> (5.4482, 6.3017)
  arc A9 (5.6227, 4.1031) -> (5.4482, 6.3017) centre (4.9486, 5.1558) ccw
  line L10 (-15.55, -20.5) -> (-15.55, -8.5)
  arc A10 (-13.55, -8.5) -> (-15.55, -8.5) centre (-14.55, -8.5) ccw
  line L11 (-13.55, -8.5) -> (-13.55, -20.5)
  arc A11 (-15.55, -20.5) -> (-13.55, -20.5) centre (-14.55, -20.5) ccw
  line L12 (9.75, -14.5) -> (9.75, -2.5)
  arc A12 (11.75, -2.5) -> (9.75, -2.5) centre (10.75, -2.5) ccw
  line L13 (11.75, -2.5) -> (11.75, -14.5)
  arc A13 (9.75, -14.5) -> (11.75, -14.5) centre (10.75, -14.5) ccw
  line L14 (-6.0958, -43.2074) -> (-4.8532, -44.45)
  line L15 (-4.8532, -44.45) -> (4.8532, -44.45)
  line L16 (4.8532, -44.45) -> (6.0958, -43.2074)
  arc A14 (10.3384, -41.45) -> (6.0958, -43.2074) centre (10.3384, -47.45) ccw
  line L17 (10.3384, -41.45) -> (13.5, -41.45)
  arc A15 (15.1961, -44.5098) -> (13.5, -41.45) centre (13.5, -43.45) ccw
  line L18 (15.1961, -44.5098) -> (7.8851, -56.2098)
  arc A16 (6.189, -57.15) -> (7.8851, -56.2098) centre (6.189, -55.15) ccw
  line L19 (6.189, -57.15) -> (-6.189, -57.15)
  arc A17 (-7.8851, -56.2098) -> (-6.189, -57.15) centre (-6.189, -55.15) ccw
  line L20 (-7.8851, -56.2098) -> (-15.1961, -44.5098)
  arc A18 (-13.5, -41.45) -> (-15.1961, -44.5098) centre (-13.5, -43.45) ccw
  line L21 (-13.5, -41.45) -> (-10.3384, -41.45)
  arc A19 (-6.0958, -43.2074) -> (-10.3384, -41.45) centre (-10.3384, -47.45) ccw
  line L22 (2.35, -23.0931) -> (2.35, -19.8578)
  arc A20 (4.253, -18.8853) -> (2.35, -19.8578) centre (3.55, -19.8578) ccw
  line L23 (4.253, -18.8853) -> (8.8217, -22.188)
  arc A21 (9.65, -23.8089) -> (8.8217, -22.188) centre (7.65, -23.8089) ccw
  line L24 (9.65, -23.8089) -> (9.65, -25.2396)
  arc A22 (6.43, -26.8244) -> (9.65, -25.2396) centre (7.65, -25.2396) ccw
  line L25 (6.43, -26.8244) -> (2.818, -24.044)
  arc A23 (2.35, -23.0931) -> (2.818, -24.044) centre (3.55, -23.0931) ccw
  line L26 (-2.35, -6.7029) -> (-2.35, -10.5206)
  arc A24 (-3.3622, -12.3724) -> (-2.35, -10.5206) centre (-4.55, -10.5206) ccw
  line L27 (-3.3622, -12.3724) -> (-4.1622, -12.8855)
  arc A25 (-7.55, -11.0338) -> (-4.1622, -12.8855) centre (-5.35, -11.0338) ccw
  line L28 (-7.55, -11.0338) -> (-7.55, -4.3629)
  arc A26 (-5.7029, -3.3523) -> (-7.55, -4.3629) centre (-6.35, -4.3629) ccw
  line L29 (-5.7029, -3.3523) -> (-3.3637, -4.8501)
  arc A27 (-2.35, -6.7029) -> (-3.3637, -4.8501) centre (-4.55, -6.7029) ccw
  line L30 (-9.75, -2.5) -> (-9.75, -14.5)
  arc A28 (-11.75, -14.5) -> (-9.75, -14.5) centre (-10.75, -14.5) ccw
  line L31 (-11.75, -14.5) -> (-11.75, -2.5)
  arc A29 (-9.75, -2.5) -> (-11.75, -2.5) centre (-10.75, -2.5) ccw
  line L32 (2.35, -10.5206) -> (2.35, -6.7029)
  arc A30 (3.3637, -4.8501) -> (2.35, -6.7029) centre (4.55, -6.7029) ccw
  line L33 (3.3637, -4.8501) -> (5.7029, -3.3523)
  arc A31 (7.55, -4.3629) -> (5.7029, -3.3523) centre (6.35, -4.3629) ccw
  line L34 (7.55, -4.3629) -> (7.55, -11.0338)
  arc A32 (4.1622, -12.8855) -> (7.55, -11.0338) centre (5.35, -11.0338) ccw
  line L35 (4.1622, -12.8855) -> (3.3622, -12.3724)
  arc A33 (2.35, -10.5206) -> (3.3622, -12.3724) centre (4.55, -10.5206) ccw
  line L36 (-6.6112, -100.95) -> (6.6112, -100.95)
  arc A34 (8.0447, -101.6962) -> (6.6112, -100.95) centre (6.6112, -102.7) ccw
  line L37 (8.0447, -101.6962) -> (8.3897, -102.1889)
  arc A35 (4.5, -105.45) -> (8.3897, -102.1889) centre (6.3028, -103.6501) ccw
  line L38 (4.5, -105.45) -> (-4.5, -105.45)
  arc A36 (-8.3897, -102.1889) -> (-4.5, -105.45) centre (-6.3028, -103.6501) ccw
  line L39 (-8.3897, -102.1889) -> (-8.0447, -101.6962)
  arc A37 (-6.6112, -100.95) -> (-8.0447, -101.6962) centre (-6.6112, -102.7) ccw
  arc A38 (2.7973, 14.2208) -> (-2.7973, 14.2208) centre (0, 7.804) ccw
  line L40 (-2.7973, 14.2208) -> (-10.9121, 10.6832)
  arc A39 (-13.7095, 10.1) -> (-10.9121, 10.6832) centre (-13.7095, 17.1) ccw
  line L41 (-13.7095, 10.1) -> (-14.75, 10.1)
  arc A40 (-14.75, 10.1) -> (-19, 2.4661) centre (-14.75, 5.1) ccw
  arc A41 (-18.55, 0.8857) -> (-19, 2.4661) centre (-21.55, 0.8857) ccw
  line L42 (-18.55, 0.8857) -> (-18.55, -26.4)
  arc A42 (-21.55, -29.4) -> (-18.55, -26.4) centre (-21.55, -26.4) ccw
  line L43 (-21.55, -29.4) -> (-30.5, -29.4)
  arc A43 (-30.5, -29.4) -> (-33.9547, -44.6156) centre (-30.5, -37.4) ccw
  arc A44 (-27.7114, -50.1961) -> (-33.9547, -44.6156) centre (-40.4322, -58.1449) ccw
  line L44 (-27.7114, -50.1961) -> (-23.2215, -57.3816)
  arc A45 (-21.55, -63.2107) -> (-23.2215, -57.3816) centre (-32.55, -63.2107) ccw
  line L45 (-21.55, -63.2107) -> (-21.55, -94.9296)
  arc A46 (-23.2215, -100.7587) -> (-21.55, -94.9296) centre (-32.55, -94.9296) ccw
  line L46 (-23.2215, -100.7587) -> (-29.5877, -110.9469)
  arc A47 (-31.6483, -113.6894) -> (-29.5877, -110.9469) centre (-46.5487, -100.3485) ccw
  line L47 (-31.6483, -113.6894) -> (-36.4601, -119.0636)
  arc A48 (-36.4601, -119.0636) -> (-27.3521, -131.7546) centre (-30.5, -124.4) ccw
  line L48 (-27.3521, -131.7546) -> (-8.3, -123.6)
  arc A49 (-4.5, -123.6) -> (-8.3, -123.6) centre (-6.4, -126.96) ccw
  line L49 (-4.5, -123.6) -> (4.5, -123.6)
  arc A50 (8.3, -123.6) -> (4.5, -123.6) centre (6.4, -126.96) ccw
  line L50 (8.3, -123.6) -> (27.3521, -131.7546)
  arc A51 (27.3521, -131.7546) -> (36.4601, -119.0636) centre (30.5, -124.4) ccw
  line L51 (36.4601, -119.0636) -> (31.6483, -113.6894)
  arc A52 (29.5877, -110.9469) -> (31.6483, -113.6894) centre (46.5487, -100.3485) ccw
  line L52 (29.5877, -110.9469) -> (23.2215, -100.7587)
  arc A53 (21.55, -94.9296) -> (23.2215, -100.7587) centre (32.55, -94.9296) ccw
  line L53 (21.55, -94.9296) -> (21.55, -63.2107)
  arc A54 (23.2215, -57.3816) -> (21.55, -63.2107) centre (32.55, -63.2107) ccw
  line L54 (23.2215, -57.3816) -> (27.7114, -50.1961)
  arc A55 (33.9547, -44.6156) -> (27.7114, -50.1961) centre (40.4322, -58.1449) ccw
  arc A56 (33.9547, -44.6156) -> (30.5, -29.4) centre (30.5, -37.4) ccw
  line L55 (30.5, -29.4) -> (21.55, -29.4)
  arc A57 (18.55, -26.4) -> (21.55, -29.4) centre (21.55, -26.4) ccw
  line L56 (18.55, -26.4) -> (18.55, 0.8857)
  arc A58 (19, 2.4661) -> (18.55, 0.8857) centre (21.55, 0.8857) ccw
  arc A59 (19, 2.4661) -> (14.75, 10.1) centre (14.75, 5.1) ccw
  line L57 (14.75, 10.1) -> (13.7095, 10.1)
  arc A60 (10.9121, 10.6832) -> (13.7095, 10.1) centre (13.7095, 17.1) ccw
  line L58 (10.9121, 10.6832) -> (2.7973, 14.2208)
  circle A61 centre (30.5, -37.4) radius 2
  circle A62 centre (15.25, -94.3) radius 2.95
  circle A63 centre (15.25, -63.8) radius 2.95
  circle A64 centre (30.5, -124.4) radius 2
  circle A65 centre (15.25, -35.5) radius 1.5
  circle A66 centre (-30.5, -37.4) radius 2
  circle A67 centre (14.75, 5.1) radius 1.5
  circle A68 centre (-15.25, -108.3) radius 1.5
  circle A69 centre (-15, -118.1) radius 2.95
  circle A70 centre (15.25, -108.3) radius 1.5
  circle A71 centre (-15.25, -94.3) radius 2.95
  circle A72 centre (15, -118.1) radius 2.95
  line L59 (5.15, -89.2) -> (-5.15, -89.2)
  arc A73 (-7.65, -86.7) -> (-5.15, -89.2) centre (-5.15, -86.7) ccw
  line L60 (-7.65, -86.7) -> (-7.65, -71.4)
  arc A74 (-5.15, -68.9) -> (-7.65, -71.4) centre (-5.15, -71.4) ccw
  line L61 (-5.15, -68.9) -> (5.15, -68.9)
  arc A75 (7.65, -71.4) -> (5.15, -68.9) centre (5.15, -71.4) ccw
  line L62 (7.65, -71.4) -> (7.65, -86.7)
  arc A76 (5.15, -89.2) -> (7.65, -86.7) centre (5.15, -86.7) ccw
  circle A77 centre (-30.5, -124.4) radius 2
  circle A78 centre (-15.25, -63.8) radius 2.95
  circle A79 centre (-15.25, -35.5) radius 1.5
  circle A80 centre (-14.75, 5.1) radius 1.5
equation "d11 = ( 29.5 / 2 ) * 1 mm"
equation "d18 = ( 37.1 / 2 ) * 1 mm"
equation "d25 = ( 30.5 / 2 ) * 1 mm"
equation "d33 = ( 43.1 / 2 ) * 1 mm"
equation "d43 = 29.8 mm - 6 mm"
equation "d63 = ( 4.7 / 2 ) * 1 mm"
equation "d67 = d63"
equation "d86 = 15.5 mm - 2 mm"

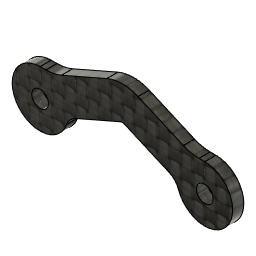
design "nose_protect"
Autodesk Fusion 360 part; units mm, degrees
sketch "Sketch1" plane through (0, 0, 0) normal (0, 0, 1) x (1, 0, 0)
  circle A0 centre (0, 0) radius 1.5
  line L0 (0, 0) -> (29.5, 0) construction
  circle A1 centre (29.5, 0) radius 1.5
  arc A2 (11.3878, -17.4724) -> (12.4, -15.6206) centre (10.2, -15.6206) ccw construction
  line L1 (3, -19.6) -> (3, -7.6) construction
  arc A3 (18.1137, -9.9501) -> (17.1, -11.8029) centre (19.3, -11.8029) ccw construction
  line L2 (29.5, 5) -> (28.4595, 5)
  line L3 (11.9527, 9.1208) -> (3.8379, 5.5832)
  arc A4 (1.2, -13.6) -> (-0.8, -13.6) centre (0.2, -13.6) ccw construction
  arc A5 (13.4019, -3.7339) -> (16.0981, -3.7339) centre (14.75, -1.6285) ccw construction
  arc A6 (33.75, -2.6339) -> (29.5, 5) centre (29.5, 0) ccw
  circle A7 centre (0, 0) radius 1.5
  line L4 (12.4, -11.8029) -> (12.4, -15.6206) construction
  arc A8 (7.2, -16.1338) -> (10.5878, -17.9855) centre (9.4, -16.1338) ccw construction
  arc A9 (17.5473, 9.1208) -> (11.9527, 9.1208) centre (14.75, 2.704) ccw
  line L5 (7.2, -16.1338) -> (7.2, -9.4629) construction
  line L6 (9.0471, -8.4523) -> (11.3863, -9.9501) construction
  arc A10 (-3.8, -4.2143) -> (-4.25, -2.6339) centre (-6.8, -4.2143) ccw construction
  arc A11 (9.3018, 1.2017) -> (9.1273, -0.9969) centre (9.8014, 0.0558) ccw construction
  line L7 (25.6621, 5.5832) -> (17.5473, 9.1208)
  line L8 (1.0405, 5) -> (0, 5)
  line L9 (15.0697, 3.4373) -> (20.1982, 1.2017) construction
  arc A12 (22.3, -9.4629) -> (20.4529, -8.4523) centre (21.1, -9.4629) ccw construction
  arc A13 (1.0405, 5) -> (3.8379, 5.5832) centre (1.0405, 12) ccw
  line L10 (17.1, -15.6206) -> (17.1, -11.8029) construction
  line L11 (9.3018, 1.2017) -> (14.4303, 3.4373) construction
  circle A14 centre (29.5, 0) radius 1.5
  arc A15 (33.75, -2.6339) -> (33.3, -4.2143) centre (36.3, -4.2143) ccw construction
  arc A16 (20.3727, -0.9969) -> (20.1982, 1.2017) centre (19.6986, 0.0558) ccw construction
  arc A17 (0, 5) -> (-4.25, -2.6339) centre (0, 0) ccw
  line L12 (18.9122, -17.9855) -> (18.1122, -17.4724) construction
  line L13 (5, -7.6) -> (5, -19.6) construction
  arc A18 (15.0697, 3.4373) -> (14.4303, 3.4373) centre (14.75, 2.704) ccw construction
  line L14 (11.3878, -17.4724) -> (10.5878, -17.9855) construction
  line L15 (18.1137, -9.9501) -> (20.4529, -8.4523) construction
  arc A19 (12.4, -11.8029) -> (11.3863, -9.9501) centre (10.2, -11.8029) ccw construction
  arc A20 (5, -7.6) -> (3, -7.6) centre (4, -7.6) ccw construction
  line L16 (24.5, -19.6) -> (24.5, -7.6) construction
  arc A21 (25.6621, 5.5832) -> (28.4595, 5) centre (28.4595, 12) ccw
  line L17 (20.3727, -0.9969) -> (16.0981, -3.7339) construction
  arc A22 (3, -19.6) -> (5, -19.6) centre (4, -19.6) ccw construction
  arc A23 (18.9122, -17.9855) -> (22.3, -16.1338) centre (20.1, -16.1338) ccw construction
  arc A24 (17.1, -15.6206) -> (18.1122, -17.4724) centre (19.3, -15.6206) ccw construction
  line L18 (13.4019, -3.7339) -> (9.1273, -0.9969) construction
  arc A25 (9.0471, -8.4523) -> (7.2, -9.4629) centre (8.4, -9.4629) ccw construction
  line L19 (26.5, -7.6) -> (26.5, -19.6) construction
  arc A26 (26.5, -7.6) -> (24.5, -7.6) centre (25.5, -7.6) ccw construction
  line L20 (22.3, -9.4629) -> (22.3, -16.1338) construction
  arc A27 (30.3, -13.6) -> (28.3, -13.6) centre (29.3, -13.6) ccw construction
  circle A28 centre (0, 0) radius 5
  circle A29 centre (29.5, 0) radius 5
  line L21 (23.2644, 0.0831) -> (15.1496, 3.6207)
  arc A30 (15.1496, 3.6207) -> (14.3504, 3.6207) centre (14.75, 2.704) ccw
  line L22 (14.3504, 3.6207) -> (6.2356, 0.0831)
  line L23 (6.2356, 0.0831) -> (4.9783, -0.4649)
  line L24 (23.2644, 0.0831) -> (24.5217, -0.4649)
  point P0 (14.75, -5.1)
  dimension "d35" = 3
  dimension "d36" = 29.5
  dimension "d37" = 3
  dimension "d38" = -6
  constraint coincident A0.centre L0.start
  constraint horizontal L0
  constraint coincident L0.end A1.centre
  constraint concentric A7 A28
  constraint coincident A10.end A28
  constraint coincident A6.start A29
  constraint tangent A15 A29
  constraint coincident A28 L23.end
  constraint collinear L22 L23
  constraint coincident A29 L24.end
  constraint collinear L21 L24
  measures "d35" diameter of A0
  measures "d36" distance of A0.centre L0.end
  measures "d37" diameter of A1
extrude "Extrude3" add sketch "Sketch1" along normal blind 2
fillet "Fillet3" radius 3 2 edges at (4.9783, -0.4649, 1) (24.5217, -0.4649, 1)

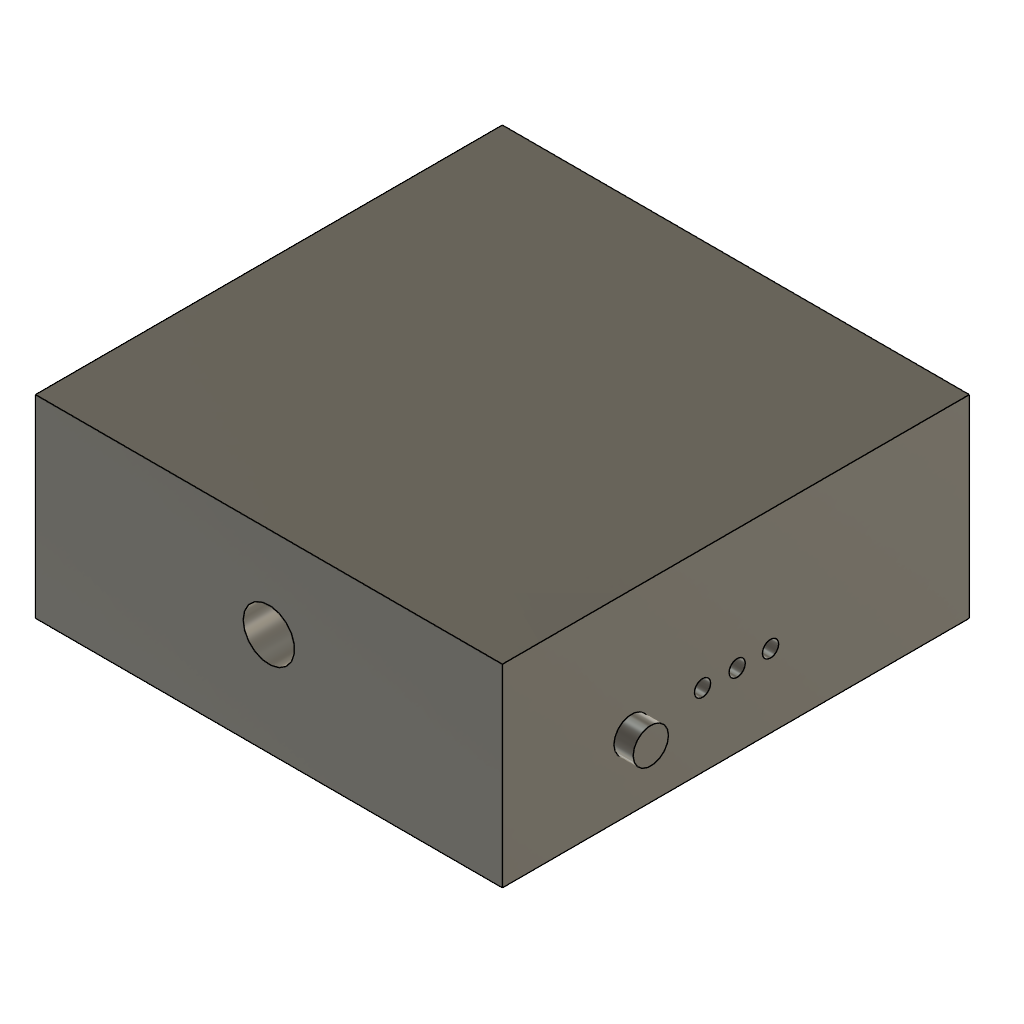
design "VTX_Envelope"
part number: 2026-09-21-19-44-39-891
Autodesk Fusion 360 part; units mm, degrees
sketch "Sketch1" plane through (0, 0, 0) normal (0, 0, 1) x (1, 0, 0)
  line L0 (-18.2, 18.2) -> (18.2, 18.2)
  line L1 (18.2, 18.2) -> (18.2, -18.2)
  line L2 (18.2, -18.2) -> (-18.2, -18.2)
  line L3 (-18.2, -18.2) -> (-18.2, 18.2)
  line L4 (-18.2, 18.2) -> (18.2, -18.2) construction
  line L5 (18.2, 18.2) -> (-18.2, -18.2) construction
  dimension "d1" = 36.4
  dimension "d2" = 36.4
  constraint horizontal L0
  constraint perpendicular L0 L1
  constraint parallel L0 L2
  constraint parallel L1 L3
  constraint coincident L4 origin
  constraint coincident L5 origin
  measures "d1" distance of L0.end L1.end
  measures "d2" distance of L1.end L2.end
extrude "Extrude1" add sketch "Sketch1" along normal blind 15.1
sketch "Sketch2" plane through (0, 0, 0) normal (0, 0, -1) x (1, 0, 0)
  line L0 (18.2, 18.2) -> (-18.2, 18.2)
  line L1 (-18.2, 18.2) -> (-18.2, -18.2)
  line L2 (-18.2, -18.2) -> (18.2, -18.2)
  line L3 (18.2, -18.2) -> (18.2, 18.2)
  circle A0 centre (-10, 10) radius 1
  circle A1 centre (10, 10) radius 1
  circle A2 centre (10, -10) radius 1
  circle A3 centre (-10, -10) radius 1
  dimension "d5" = 2
  dimension "d6" = 2
  dimension "d7" = 2
  dimension "d8" = 2
  dimension "d9" = 10
  dimension "d10" = 10
  dimension "d11" = 10
  dimension "d12" = 10
  dimension "d13" = 10
  dimension "d14" = 10
  dimension "d15" = 10
  dimension "d16" = 10
  measures "d5" diameter of A0
  measures "d6" diameter of A1
  measures "d7" diameter of A2
  measures "d8" diameter of A3
  measures "d9" horizontal distance of origin A0.centre
  measures "d10" vertical distance of origin A0.centre
  measures "d11" vertical distance of origin A2.centre
  measures "d12" horizontal distance of origin A2.centre
  measures "d13" vertical distance of origin A1.centre
  measures "d14" horizontal distance of origin A1.centre
  measures "d15" vertical distance of origin A3.centre
  measures "d16" horizontal distance of origin A3.centre